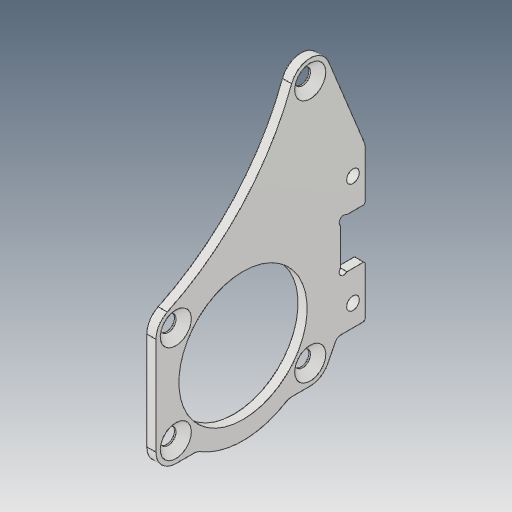
# Autodesk Inventor part: tab_pitch_out
Saved by Autodesk Inventor 2019.4 (Build 234330000, 330)
## iProperties
Created: 2018-04-26
Part Number: tab_pitch_out
Material: 一般
Document SubType Name: Modeling
Designer: cmflab
Density: 1 g/cm^3
Appearance: 滑らか - 白
Mass: 1.07958 g
Surface Area: 18.5636 cm^2
Volume: 1.07958 cm^3
Author: cmflab
Autodesk Inventor part; units mm, degrees
ref_plane "YZ Plane" through (0, 0, 0) normal (1, 0, 0) x (0, 1, 0)
ref_plane "XZ Plane" through (0, 0, 0) normal (0, 1, 0) x (-1, 0, 0)
ref_plane "XY Plane" through (0, 0, 0) normal (0, 0, 1) x (1, 0, 0)
sketch "スケッチ1" plane through (0, 0, 0) normal (1, 0, 0) x (0, 1, 0)
  line L0 (12.5, 2) -> (-12.5, 2) construction
  line L1 (-12.5, 2) -> (-12.5, -2)
  line L2 (-12.5, -2) -> (-4.05, -2)
  line L3 (12.5, -2) -> (12.5, 2) construction
  line L4 (0, 0) -> (0, 21.2341) construction
  line L5 (0, 0) -> (25.6299, 0) construction
  circle A0 centre (9, 0) radius 1.05
  circle A1 centre (-9, 0) radius 1.05
  line L6 (-17.25, 7) -> (-17.25, 9.9571)
  line L7 (-14, 32.25) -> (2, 32.25)
  arc A2 (4.9363, 30.393) -> (27.1329, 10.0462) centre (41.0759, 47.5374) ccw
  arc A3 (-17.25, 7) -> (-15.4518, 4.0923) centre (-14, 7) ccw
  arc A4 (-14, 32.25) -> (-17.25, 29) centre (-14, 29) ccw
  arc A5 (4.9363, 30.393) -> (2, 32.25) centre (2, 29) ccw
  circle A6 centre (2, 29) radius 1.3
  circle A7 centre (-14, 29) radius 1.3
  circle A8 centre (-14, 7) radius 1.3
  circle A9 centre (26, 7) radius 1.3
  arc A10 (27.2246, 3.9895) -> (27.1329, 10.0462) centre (26, 7) ccw
  line L8 (2, 29) -> (-14, 29) construction
  line L9 (-6, 29) -> (-6, 7) construction
  line L10 (-6, 7) -> (-14, 7) construction
  circle A11 centre (-6, 18) radius 10.5
  arc A12 (-17.5403, 25.0051) -> (-17.5403, 10.9949) centre (-6, 18) ccw
  line L11 (-17.25, 10.5376) -> (-17.25, 25.4624) construction
  line L12 (-17.25, 26.0429) -> (-17.25, 29)
  arc A13 (-17.5403, 25.0051) -> (-17.25, 26.0429) centre (-19.25, 26.0429) ccw
  arc A14 (-17.25, 9.9571) -> (-17.5403, 10.9949) centre (-19.25, 9.9571) ccw
  line L13 (-6, 18) -> (10, 18) construction
  line L14 (27.2246, 3.9895) -> (12.5, -2)
  line L15 (-4.05, -2) -> (-4.05, 0.9893)
  line L16 (-4.05, 2.05) -> (-2.9893, 2.05) construction
  line L17 (4.05, 2.05) -> (4.05, 0.9893) construction
  line L18 (-4.05, -2) -> (4.05, -2) construction
  line L19 (4.05, -2) -> (12.5, -2)
  arc A15 (4.05, 0.9893) -> (2.9893, 2.05) centre (3.5197, 1.5197) ccw
  line L20 (4.05, 0.9893) -> (4.05, -2)
  line L21 (2.9893, 2.05) -> (4.05, 2.05) construction
  line L22 (-2.9893, 2.05) -> (2.9893, 2.05)
  line L23 (-4.05, 0.9893) -> (-4.05, 2.05) construction
  arc A16 (-2.9893, 2.05) -> (-4.05, 0.9893) centre (-3.5197, 1.5197) ccw
  line L24 (3.5197, 1.5197) -> (4.05, 2.05) construction
  line L25 (-3.5197, 1.5197) -> (-4.05, 2.05) construction
  line L26 (-12.5, -2) -> (-12.5, 2) construction
  arc A17 (-12.5, 2) -> (-13.0533, 2.8947) centre (-13.5, 2) ccw
  line L27 (-15.4518, 4.0923) -> (-13.0533, 2.8947)
  point P0 (4.1125, 32.25)
  point P1 (16.6739, 3.086)
  dimension "d2" = 18
  dimension "d3" = 2.1
  dimension "d7" = 16
  dimension "d8" = 2.6
  dimension "d13" = 3.25
  dimension "d14" = 21
  dimension "d15" = 40
  dimension "d17" = 40
  dimension "d18" = 6
  dimension "d21" = 3
  dimension "d22" = 2
  dimension "d27" = 18
  dimension "d28" = 22
  dimension "d30" = 8.1
  dimension "d31" = 4
  dimension "d32" = 4.05
  dimension "d33" = 0.75
  dimension "d34" = 45
  dimension "d35" = 45
  dimension "d36" = 1
  constraints: 56 end point, 27 point on circle, 18 centre point, 18 tangent, 10 vertical, 9 equal radius, 9 point on line, 7 horizontal, 5 perpendicular, 4 coincident, 4 parallel, 3 midpoint, 1 concentric, 1 horizontal alignment, 1 symmetric about line, 5 other
  measures "d2" distance of A1.centre A0.centre
  measures "d3" diameter of A0
  measures "d7" distance of A4.centre A5.centre
  measures "d8" diameter of A9
  measures "d13" radius of A5
  measures "d14" diameter of A11
  measures "d15" radius of A2
  measures "d17" distance of A3.centre A9.centre
  measures "d18" distance between parallel lines of L9 L4
  measures "d21" radial gap between concentric circles of A12 A11
  measures "d22" radius of A13
  measures "d27" distance from line of L5 A11.centre
  measures "d28" distance between parallel lines of L10 L8
  measures "d30" diameter of L15 L4
  measures "d31" distance between parallel lines of L0 L19
  measures "d32" distance between parallel lines of L18 L16
  measures "d33" radius of A15
  measures "d34" angle of L24 L21
  measures "d35" angle of L25 L16
  measures "d36" radius of A17
extrude "押し出し1" add sketch "スケッチ1" along normal blind 1.5
chamfer "面取り1" distance 0.25 angle 45 4 edges at (0.75, -12.5, -2) (0.75, -4.05, -2) (0.75, 4.05, -2) (0.75, 12.5, -2)
chamfer "面取り2" distance 1.25 angle 45 4 edges at (1.5, 24.7, 7) (1.5, 0.7, 29) (1.5, -15.3, 29) (1.5, -15.3, 7)
